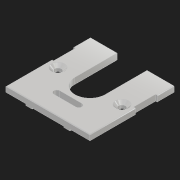
# Autodesk Inventor part: Plaque de maintient
Saved by Autodesk Inventor 2017 (Build 210142000, 142)
## iProperties
Company: FABLAB Frenchmakers
Part Number: Plaque de maintient
Material: ----------
Document SubType Name: Modeling
Designer: FABLAB Frenchmakers
Density: 7.86 g/cm^3
Appearance: Métal
Mass: 30.8751 g
Surface Area: 34.3395 cm^2
Volume: 3.92813 cm^3
Project: 1420 Vauban 3D XL
Catalog Web Link: http://frenchmakers.com/
Stock Number: 1420-05-16
Autodesk Inventor part; units mm, degrees
ref_plane "YZ Plane" through (0, 0, 0) normal (1, 0, 0) x (0, 1, 0)
ref_plane "XZ Plane" through (0, 0, 0) normal (0, 1, 0) x (-1, 0, 0)
ref_plane "XY Plane" through (0, 0, 0) normal (0, 0, 1) x (1, 0, 0)
sketch "Esquisse1" plane through (0, 0, 0) normal (0, 0, 1) x (1, 0, 0)
  line L0 (-21, -21) -> (21, -21)
  line L1 (21, -21) -> (21, 21)
  line L2 (21, 21) -> (-21, 21)
  line L3 (-21, 21) -> (-21, -21)
  point P0 (0, 0)
  dimension "d0" = 42
  dimension "d1" = 42
  dimension "d2" = 21
  dimension "d3" = 21
  constraints: 8 end point, 3 perpendicular, 1 horizontal
  measures "d0" distance between parallel lines of L0 L2
  measures "d1" distance between parallel lines of L3 L1
  measures "d2" distance from line of point (0, 0) L2
  measures "d3" distance from line of point (0, 0) L1
extrude "Extrusion1" add sketch "Esquisse1" along normal blind 3
sketch "Esquisse2" plane through (0, 0, 3) normal (0, 0, 1) x (1, 0, 0)
  line L0 (21, 1.8) -> (20, 1.8)
  line L1 (20, 1.8) -> (20, 12.8)
  line L2 (20, 12.8) -> (21, 12.8)
  line L3 (21, 12.8) -> (21, 1.8)
  line L4 (-21, 1.8) -> (-20, 1.8)
  line L5 (-20, 1.8) -> (-20, 12.8)
  line L6 (-20, 12.8) -> (-21, 12.8)
  line L7 (-21, 12.8) -> (-21, 1.8)
  line L8 (21, 21) -> (-21, 21) projected
  line L9 (-21, 21) -> (-21, -21) projected
  line L10 (21, -21) -> (21, 21) projected
  point P0 (0, 0)
  dimension "d6" = 40
  dimension "d7" = 20
  dimension "d8" = 11
  dimension "d9" = 8.2
  constraints: 16 end point, 4 collinear, 4 parallel, 2 horizontal, 2 perpendicular
  measures "d6" distance between parallel lines of L1 L5
  measures "d7" distance from line of point (0, 0) L1
  measures "d8" distance of L4.end L5.end
  measures "d9" distance between parallel lines of L8 L6
extrude "Extrusion2" cut sketch "Esquisse2" against normal through all
sketch "Esquisse3" plane through (0, 0, 3) normal (0, 0, 1) x (1, 0, 0)
  line L0 (7.5, 0) -> (7.5, 21)
  line L1 (7.5, 21) -> (-7.5, 21)
  line L2 (-7.5, 21) -> (-7.5, 0)
  line L3 (21, 21) -> (-21, 21) projected
  arc A0 (-7.5, 0) -> (7.5, 0) centre (0, 0) ccw
  line L4 (-5.5, -11.1) -> (5.5, -11.1) construction
  line L5 (-5.5, -12.6) -> (5.5, -12.6)
  line L6 (5.5, -9.6) -> (-5.5, -9.6)
  arc A1 (-5.5, -9.6) -> (-5.5, -12.6) centre (-5.5, -11.1) ccw
  arc A2 (5.5, -12.6) -> (5.5, -9.6) centre (5.5, -11.1) ccw
  line L7 (-21, -21) -> (21, -21) projected
  point P0 (0, 0)
  point P1 (0, -11.1)
  dimension "d12" = 15
  dimension "d13" = 7.5
  dimension "d14" = 21
  dimension "d15" = 3
  dimension "d16" = 14
  dimension "d17" = 8.4
  constraints: 14 end point, 6 point on circle, 6 tangent, 3 centre point, 2 parallel, 1 collinear, 1 horizontal, 1 midpoint, 1 vertical, 1 vertical alignment
  measures "d12" distance between parallel lines of L0 L2
  measures "d13" distance from line of point (0, 0) L0
  measures "d14" distance from line of L3 A0.centre
  measures "d15" distance between parallel lines of L6 L5
  measures "d17" distance between parallel lines of L7 L5
extrude "Extrusion3" cut sketch "Esquisse3" against normal through all
sketch "Esquisse4" plane through (0, 0, 0) normal (0, 0, -1) x (-1, 0, 0)
  line L0 (21, -21) -> (-21, -21) projected
  line L1 (-11, -21) -> (-7.95, -21)
  line L2 (-7.95, -21) -> (-7.95, 21)
  line L3 (-7.95, 21) -> (-11, 21)
  line L4 (-11, 21) -> (-11, -21)
  line L5 (7.95, -21) -> (11, -21)
  line L6 (11, -21) -> (11, 21)
  line L7 (11, 21) -> (7.95, 21)
  line L8 (7.95, 21) -> (7.95, -21)
  line L9 (7.5, 21) -> (21, 21) projected
  point P0 (0, 0)
  dimension "d20" = 3.05
  dimension "d21" = 3.05
  dimension "d22" = 15.9
  dimension "d23" = 7.95
  constraints: 16 end point, 4 parallel, 3 point on line, 2 horizontal, 2 perpendicular, 1 collinear
  measures "d20" distance between parallel lines of L8 L6
  measures "d21" distance between parallel lines of L4 L2
  measures "d22" distance between parallel lines of L8 L2
  measures "d23" distance from line of point (0, 0) L8
extrude "Extrusion4" add sketch "Esquisse4" along normal blind 0.5
chamfer "Chanfrein1" distance 0.25 angle 45 12 edges at (16, 21, 0) (21, 16.9, 0) (16, -21, 0) (-16, -21, 0) (-21, -9.6, 0) (-16, 21, 0) (21, -9.6, 0) (-21, 16.9, 3) (-21, -9.6, 3) (0, -21, 3) (21, -9.6, 3) (21, 16.9, 3)
sketch "Esquisse5" plane through (0, 0, 3) normal (0, 0, 1) x (1, 0, 0)
  line L0 (-7.5, 21) -> (-20.75, 21) projected
  point P0 (0, 0)
  point P1 (-16, 0)
  point P2 (16, 0)
  dimension "d29" = 32
  dimension "d30" = 16
  dimension "d31" = 21
  constraints: 1 horizontal alignment
  measures "d29" distance of point (-16, 0) point (16, 0)
  measures "d30" distance of point (0, 0) point (-16, 0)
  measures "d31" distance from line of L0 point (-16, 0)
hole "Perçage1" at (-16, 0, 3) at (16, 0, 3) direction (0, 0, -1) diameter 3.5 end through all countersink diameter 6.5 countersink angle 90
equation "\"d2\" = 0.5 * d0"
equation "\"d3\" = 0.5 * d1"
equation "\"d7\" = 0.5 * d6"
equation "\"d13\" = 0.5 * d12"
equation "\"d21\" = d20"
equation "\"d23\" = 0.5 * d22"
equation "\"d30\" = 0.5 * d29"
